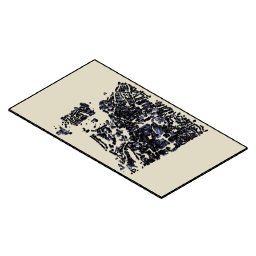
FlaecheStadtmodell (Autodesk Fusion 360 design; units mm, degrees)
Autodesk Fusion 360 part; units mm, degrees
sketch "Skizze1" plane through (0, 0, 0) normal (0, 1, 0) x (1, 0, 0)
  line L0 (0, 0) -> (1422.2222, 0)
  line L1 (1422.2222, 0) -> (1422.2222, -800)
  line L2 (1422.2222, -800) -> (0, -800)
  line L3 (0, -800) -> (0, 0)
  line L4 (711.1111, 0) -> (711.1111, -800) construction
  line L5 (1111.1111, 0) -> (1111.1111, -800)
  line L6 (311.1111, 0) -> (311.1111, -800)
  dimension "d1" = 1422.2222
  dimension "d2" = 800
  dimension "d5" = 400
  dimension "d6" = 311.1111
  constraint horizontal L0
  constraint vertical L1
  constraint horizontal L2
  constraint vertical L3
  constraint coincident L0.start L3.end
  constraint midpoint L0 L4.start
  constraint midpoint L2 L4.end
  constraint coincident L0 L5.start
  constraint coincident L2 L5.end
  constraint perpendicular L2 L5
  constraint coincident L0 L6.start
  constraint coincident L2 L6.end
  constraint perpendicular L2 L6
  constraint symmetric L4 L5 L6
  measures "d1" distance of L0.start L0.end
  measures "d2" distance of L0.start L2.end
  measures "d5" distance of L4 L6
  measures "d6" distance of L3 L6
other "Grundnetzelement1"
other "Maßstab1"
other "Ändern1"
other "Ändern2"
extrude "Extrusion1" add sketch "Skizze1" against normal blind 10
equation "d1 = Laenge"
equation "d2 = Hoehe"
equation "Hoehe = 800 mm"
equation "Laenge = ( Hoehe / 9 ) * 16"
equation "d5 = Hoehe / 2"
